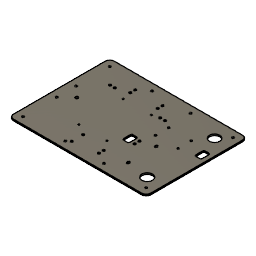
layer3_plate_v0_1 (Autodesk Fusion 360 design; units mm, degrees)
part number: 2026-05-30-19-40-51-836
Autodesk Fusion 360 part; units mm, degrees
box "长方体基本要素1" add length 209.6 width 285 height 3 placed x (0, 0, 1) y (1, 0, 0) z (0, 1, 0) at (0, 0, 0)
sketch "草图2" plane through (0, 3, 0) normal (0, 1, 0) x (-1, 0, 0)
  line L0 (0, 209.6) -> (-285, 209.6)
  line L1 (-285, 209.6) -> (-285, 0)
  line L2 (-285, 0) -> (0, 0)
  line L3 (0, 0) -> (0, 209.6)
  line L4 (-285, 104.8) -> (0, 104.8) construction
  line L5 (-142.5, 0) -> (-142.5, 209.6) construction
  circle A0 centre (-252.0096, 174.6) radius 11.05
  circle A1 centre (-252.0096, 35) radius 10.68
  circle A2 centre (-252.0096, 35) radius 14.275
  line L6 (-252.0096, 189.6) -> (-265, 182.1)
  line L7 (-265, 182.1) -> (-265, 167.1)
  line L8 (-265, 167.1) -> (-252.0096, 159.6)
  line L9 (-252.0096, 159.6) -> (-239.0192, 167.1)
  line L10 (-239.0192, 167.1) -> (-239.0192, 182.1)
  line L11 (-239.0192, 182.1) -> (-252.0096, 189.6)
  line L12 (-70.6, 54.8) -> (-148.4, 54.8)
  line L13 (-149, 55.4) -> (-149, 154.2)
  line L14 (-148.4, 154.8) -> (-70.6, 154.8)
  line L15 (-70, 154.2) -> (-70, 55.4)
  line L16 (-70, 54.8) -> (-149, 154.8) construction
  line L17 (-149, 54.8) -> (-70, 154.8) construction
  line L18 (-179, 59.87) -> (-239.07, 59.87)
  line L19 (-239.07, 59.87) -> (-239.07, 94.8)
  line L20 (-239.07, 94.8) -> (-179, 94.8)
  line L21 (-179, 94.8) -> (-179, 59.87)
  line L22 (0, 72.3) -> (-30, 72.3)
  line L23 (-30, 72.3) -> (-30, 137.3)
  line L24 (-30, 137.3) -> (0, 137.3)
  arc A3 (-70.6, 54.8) -> (-70, 55.4) centre (-70.6, 55.4) ccw
  arc A4 (-149, 55.4) -> (-148.4, 54.8) centre (-148.4, 55.4) ccw
  arc A5 (-70, 154.2) -> (-70.6, 154.8) centre (-70.6, 154.2) ccw
  arc A6 (-148.4, 154.8) -> (-149, 154.2) centre (-148.4, 154.2) ccw
  circle A7 centre (-270, 194.6) radius 2.15
  circle A8 centre (-270, 15) radius 2.15
  circle A9 centre (-15, 15) radius 2.15
  circle A10 centre (-15, 194.6) radius 2.15
  circle A11 centre (-182.5, 15) radius 2.15
  circle A12 centre (-102.5, 15) radius 2.15
  circle A13 centre (-102.5, 194.6) radius 2.15
  circle A14 centre (-182.5, 194.6) radius 2.15
  line L25 (-15, 72.3) -> (-15, 137.3) construction
  circle A15 centre (-15, 84.8) radius 2.15
  circle A16 centre (-15, 124.8) radius 2.15
  line L26 (-109.5, 54.8) -> (-109.5, 154.8) construction
  circle A17 centre (-87, 58.8) radius 1.6
  circle A18 centre (-145, 58.8) radius 1.6
  circle A19 centre (-87, 150.8) radius 1.6
  circle A20 centre (-145, 150.8) radius 1.6
  circle A21 centre (-232.375, 63.695) radius 1.99
  line L27 (-209.035, 59.87) -> (-209.035, 94.8) construction
  line L28 (-239.07, 77.335) -> (-179, 77.335) construction
  circle A22 centre (-232.375, 90.975) radius 1.99
  circle A23 centre (-185.695, 63.695) radius 1.99
  circle A24 centre (-185.695, 90.975) radius 1.99
  line L29 (-273, 68.335) -> (-265, 68.335)
  line L30 (-263, 70.335) -> (-263, 84.335)
  line L31 (-265, 86.335) -> (-273, 86.335)
  line L32 (-275, 84.335) -> (-275, 70.335)
  arc A25 (-265, 68.335) -> (-263, 70.335) centre (-265, 70.335) ccw
  arc A26 (-275, 70.335) -> (-273, 68.335) centre (-273, 70.335) ccw
  arc A27 (-263, 84.335) -> (-265, 86.335) centre (-265, 84.335) ccw
  arc A28 (-273, 86.335) -> (-275, 84.335) centre (-273, 84.335) ccw
  circle A29 centre (-109.5, 164.8) radius 1.75
  circle A30 centre (-109.5, 188.3) radius 1.75
  line L33 (-109.5, 188.3) -> (-109.5, 164.8) construction
  line L34 (-109.5, 176.55) -> (-126.71, 176.55) construction
  circle A31 centre (-169, 54.8) radius 1.75
  circle A32 centre (-159, 54.8) radius 1.75
  circle A33 centre (-139.6536, 30.484) radius 1.75
  circle A34 centre (-139.6536, 40.484) radius 1.75
  circle A35 centre (-82.9945, 30.484) radius 1.75
  circle A36 centre (-82.9945, 40.484) radius 1.75
  line L35 (-139.6536, 30.484) -> (-139.6536, 40.484) construction
  line L36 (-138.8486, 35.484) -> (-115.3178, 35.484) construction
  circle A37 centre (-58.3945, 48.0031) radius 1.75
  circle A38 centre (-48.3945, 48.0031) radius 1.75
  circle A39 centre (-264, 157.9214) radius 1.75
  circle A40 centre (-252.0096, 174.6) radius 22.75
  line L37 (-273, 68.335) -> (-265, 68.335)
  line L38 (-275, 84.335) -> (-275, 70.335)
  line L39 (-265, 86.335) -> (-273, 86.335)
  line L40 (-263, 70.335) -> (-263, 84.335)
  arc A41 (-273, 86.335) -> (-275, 84.335) centre (-273, 84.335) ccw
  arc A42 (-265, 68.335) -> (-263, 70.335) centre (-265, 70.335) ccw
  arc A43 (-263, 84.335) -> (-265, 86.335) centre (-265, 84.335) ccw
  arc A44 (-275, 70.335) -> (-273, 68.335) centre (-273, 70.335) ccw
  circle A45 centre (-158.9706, 171.55) radius 1.75
  circle A46 centre (-158.9706, 181.55) radius 1.75
  line L41 (-222.2263, 163.8539) -> (-190.2263, 163.8539)
  line L42 (-190.2263, 163.8539) -> (-190.2263, 113.8539)
  line L43 (-190.2263, 113.8539) -> (-222.2263, 113.8539)
  line L44 (-222.2263, 113.8539) -> (-222.2263, 163.8539)
  line L45 (-206.2263, 163.8539) -> (-206.2263, 166.8539) construction
  line L46 (-206.2263, 166.8539) -> (-206.2263, 168.7439) construction
  line L47 (-208.3763, 166.8539) -> (-208.3763, 168.7439)
  line L48 (-204.0763, 168.7439) -> (-204.0763, 166.8539)
  arc A47 (-204.0763, 168.7439) -> (-208.3763, 168.7439) centre (-206.2263, 168.7439) ccw
  arc A48 (-208.3763, 166.8539) -> (-204.0763, 166.8539) centre (-206.2263, 166.8539) ccw
  line L49 (-222.2263, 138.8539) -> (-190.2263, 138.8539) construction
  arc A49 (-204.0763, 110.8539) -> (-208.3763, 110.8539) centre (-206.2263, 110.8539) ccw
  line L50 (-206.2263, 110.8539) -> (-206.2263, 108.9639) construction
  line L51 (-208.3763, 110.8539) -> (-208.3763, 108.9639)
  arc A50 (-208.3763, 108.9639) -> (-204.0763, 108.9639) centre (-206.2263, 108.9639) ccw
  line L52 (-204.0763, 108.9639) -> (-204.0763, 110.8539)
  line L53 (-161, 113.8539) -> (-169, 113.8539)
  line L54 (-171, 115.8539) -> (-171, 129.8539)
  line L55 (-169, 131.8539) -> (-161, 131.8539)
  line L56 (-159, 129.8539) -> (-159, 115.8539)
  arc A51 (-161, 113.8539) -> (-159, 115.8539) centre (-161, 115.8539) ccw
  arc A52 (-171, 115.8539) -> (-169, 113.8539) centre (-169, 115.8539) ccw
  arc A53 (-169, 131.8539) -> (-171, 129.8539) centre (-169, 129.8539) ccw
  arc A54 (-159, 129.8539) -> (-161, 131.8539) centre (-161, 129.8539) ccw
  line L57 (-171, 122.8539) -> (-159, 122.8539) construction
  circle A55 centre (-179.3475, 117.8539) radius 1.75
  circle A56 centre (-179.3475, 127.8539) radius 1.75
  line L58 (-124, 124.8) -> (-144, 124.8)
  line L59 (-144, 124.8) -> (-144, 144.8)
  line L60 (-144, 144.8) -> (-124, 144.8)
  line L61 (-124, 144.8) -> (-124, 124.8)
  circle A57 centre (-125.75, 15) radius 3.25
  circle A58 centre (-125.75, 194.6) radius 3.25
  point P0 (-252.0096, 174.6)
  point P1 (-109.5, 104.8)
  point P2 (-182.5, 194.6)
  point P3 (-275, 68.335)
  point P4 (-263, 68.335)
  point P5 (-275, 86.335)
  point P6 (-275, 68.335)
  point P7 (-263, 68.335)
  point P8 (-275, 86.335)
  point P9 (-159, 113.8539)
  point P10 (-171, 113.8539)
  point P11 (-159, 131.8539)
  dimension "d8" = 22.1
  dimension "d9" = 21.36
  dimension "d10" = 28.55
  dimension "d11" = 15
  dimension "d12" = 20
  dimension "d14" = 79
  dimension "d15" = 100
  dimension "d18" = 34.93
  dimension "d19" = 60.07
  dimension "d20" = 30
  dimension "d21" = 65
  dimension "d22" = 40
  dimension "d33" = 0.6
  dimension "d34" = 0.6
  dimension "d35" = 0.6
  dimension "d36" = 0.6
  dimension "d47" = 4.3
  dimension "d48" = 15
  dimension "d49" = 15
  dimension "d50" = 4.3
  dimension "d51" = 15
  dimension "d52" = 80
  dimension "d53" = 4.3
  dimension "d54" = 40
  dimension "d55" = 3.2
  dimension "d56" = 4
  dimension "d57" = 3.2
  dimension "d58" = 4
  dimension "d59" = 4
  dimension "d60" = 58
  dimension "d61" = 3.98
  dimension "d62" = 27.28
  dimension "d63" = 46.68
  dimension "d75" = 12
  dimension "d76" = 18
  dimension "d79" = 10
  dimension "d81" = 2
  dimension "d82" = 2
  dimension "d83" = 2
  dimension "d84" = 2
  dimension "d99" = 35
  dimension "d100" = 3.5
  dimension "d101" = 3.5
  dimension "d102" = 23.5
  dimension "d103" = 10
  dimension "d107" = 3.5
  dimension "d108" = 10
  dimension "d109" = 10
  dimension "d110" = 3.5
  dimension "d111" = 10
  dimension "d112" = 10
  dimension "d113" = 3.5
  dimension "d114" = 10
  dimension "d123" = 30
  dimension "d124" = 45.5
  dimension "d144" = 12
  dimension "d145" = 18
  dimension "d146" = 2
  dimension "d147" = 2
  dimension "d148" = 2
  dimension "d149" = 2
  dimension "d185" = 3.5
  dimension "d186" = 3.5
  dimension "d187" = 10
  dimension "d210" = 32
  dimension "d211" = 50
  dimension "d212" = 3
  dimension "d214" = 1.89
  dimension "d215" = 2.15
  dimension "d218" = 12
  dimension "d219" = 18
  dimension "d220" = 2
  dimension "d223" = 10
  dimension "d224" = 3.5
  dimension "d225" = 3.5
  dimension "d226" = 10
  dimension "d227" = 9
  dimension "d248" = 20
  dimension "d249" = 20
  dimension "d250" = 10
  dimension "d251" = 5
  dimension "d252" = 6.5
  dimension "d253" = 23.25
  dimension "d254" = 15
  constraint midpoint L1 L4.start
  constraint midpoint L3 L4.end
  constraint midpoint L2 L5.start
  constraint midpoint L0 L5.end
  constraint concentric A1 A2
  constraint coincident P0 A0.centre
  constraint symmetric L4 P0 A1.centre
  constraint parallel L1 L7
  constraint horizontal L12
  constraint perpendicular L12 L13
  constraint parallel L12 L14
  constraint parallel L13 L15
  constraint coincident L16 P1
  constraint coincident L17 P1
  constraint horizontal L18
  constraint vertical L19
  constraint horizontal L20
  constraint vertical L21
  constraint coincident L4 P1
  constraint coincident L3 L22.start
  constraint perpendicular L3 L22
  constraint perpendicular L4 L23
  constraint coincident L3 L24.end
  constraint perpendicular L3 L24
  constraint symmetric L4 L22 L24
  constraint coincident L16.start L15
  constraint coincident L16.start L12
  constraint tangent L15 A3
  constraint tangent L12 A3
  constraint coincident L17.start L12
  constraint coincident L17.start L13
  constraint tangent L12 A4
  constraint tangent L13 A4
  constraint coincident L17.end L14
  constraint coincident L17.end L15
  constraint tangent L14 A5
  constraint tangent L15 A5
  constraint coincident L16.end L14
  constraint coincident L16.end L13
  constraint tangent L14 A6
  constraint tangent L13 A6
  constraint symmetric L4 A7 A8
  constraint symmetric L5 A7 A10
  constraint symmetric L5 A8 A9
  constraint symmetric L5 A11 A12
  constraint symmetric L4 A11.centre P2
  constraint symmetric L4 A12 A13
  constraint symmetric L4 A11 A14
  constraint midpoint L22 L25.start
  constraint midpoint L24 L25.end
  constraint coincident L25 A15.centre
  constraint symmetric L4 A15 A16
  constraint midpoint L12 L26.start
  constraint midpoint L14 L26.end
  constraint symmetric L4 A17 A19
  constraint symmetric L4 A18 A20
  constraint midpoint L18 L27.start
  constraint midpoint L20 L27.end
  constraint midpoint L19 L28.start
  constraint midpoint L21 L28.end
  constraint symmetric A21 L28 A22
  constraint symmetric A21 L27 A23
  constraint symmetric L27 A22 A24
  constraint horizontal L29
  constraint vertical L30
  constraint horizontal L31
  constraint vertical L32
  constraint symmetric L28 L29 L31
  constraint coincident P7 L30
  constraint tangent L30 A25
  constraint tangent L29 A25
  constraint coincident P6 L32
  constraint tangent L32 A26
  constraint tangent L29 A26
  constraint tangent L31 A27
  constraint tangent L30 A27
  constraint coincident P8 L31
  constraint coincident P8 L32
  constraint tangent L31 A28
  constraint tangent L32 A28
  constraint vertical A29.centre A30.centre
  constraint coincident A30.centre L33.start
  constraint coincident A29.centre L33.end
  constraint midpoint L33 L34.start
  constraint perpendicular L33 L34
  constraint equal A31 A32
  constraint horizontal L12.end A32.centre
  constraint horizontal A31.centre A32.centre
  constraint equal A35 A36
  constraint equal A34 A36
  constraint equal A33 A36
  constraint vertical A33.centre A34.centre
  constraint vertical A35.centre A36.centre
  constraint coincident A33.centre L35.start
  constraint coincident A34.centre L35.end
  constraint perpendicular L35 L36
  constraint symmetric A33.centre A34.centre L36
  constraint symmetric A35.centre A36.centre L36
  constraint equal A37 A38
  constraint horizontal A37.centre A38.centre
  constraint concentric A0 A40
  constraint horizontal L37
  constraint vertical L40
  constraint horizontal L39
  constraint vertical L38
  constraint coincident P7 L40
  constraint tangent L40 A42
  constraint tangent L37 A42
  constraint coincident P6 L38
  constraint tangent L38 A44
  constraint tangent L37 A44
  constraint tangent L39 A43
  constraint tangent L40 A43
  constraint coincident P8 L39
  constraint coincident P8 L38
  constraint tangent L39 A41
  constraint tangent L38 A41
  constraint vertical A45.centre A46.centre
  constraint symmetric L34 A45.centre A46.centre
  constraint horizontal L41
  constraint vertical L42
  constraint horizontal L43
  constraint vertical L44
  constraint midpoint L41 L45.start
  constraint perpendicular L41 L45
  constraint coincident L45.end L46.start
  constraint parallel L45 L46
  constraint coincident L46.end A47.centre
  constraint equal A47 A48
  constraint tangent L48 A48
  constraint tangent L48 A47
  constraint tangent L47 A48
  constraint tangent L47 A47
  constraint midpoint L44 L49.start
  constraint midpoint L42 L49.end
  constraint symmetric L45.end L49 A49.centre
  constraint symmetric L46.end L49 L50.end
  constraint symmetric L47.start L49 A49.end
  constraint symmetric L47.end L49 L51.end
  constraint symmetric L48.start L49 A50.end
  constraint symmetric L48.end L49 A49.start
  constraint symmetric A47 L49 A50
  constraint symmetric A48 L49 A49
  constraint horizontal L53
  constraint vertical L54
  constraint horizontal L55
  constraint vertical L56
  constraint coincident P9 L56
  constraint coincident P9 L53
  constraint tangent L56 A51
  constraint tangent L53 A51
  constraint coincident P10 L54
  constraint coincident P10 L53
  constraint tangent L54 A52
  constraint tangent L53 A52
  constraint tangent L55 A53
  constraint tangent L54 A53
  constraint equal A52 A53
  constraint coincident P11 L55
  constraint coincident P11 L56
  constraint tangent L55 A54
  constraint tangent L56 A54
  constraint equal A51 A52
  constraint equal A51 A54
  constraint midpoint L54 L57.start
  constraint midpoint L56 L57.end
  constraint symmetric L57 A55.centre A56.centre
  constraint horizontal L58
  constraint vertical L59
  constraint horizontal L60
  constraint vertical L61
  constraint symmetric L4 A57 A58
  measures "d8" diameter of A0
  measures "d9" diameter of A1
  measures "d10" diameter of A2
  measures "d11" distance of L6.start L10.end
  measures "d12" distance of L1 L7
  measures "d14" distance of L16.end L17.end
  measures "d15" distance of L17.start L16.end
  measures "d18" distance of L18.start L20.end
  measures "d19" distance of L18.start L18.end
  measures "d20" distance of L22.start L22.end
  measures "d21" distance of L22.end L23.end
  measures "d22" distance of L15 L23
  measures "d33" radius of A3
  measures "d34" radius of A4
  measures "d35" radius of A5
  measures "d36" radius of A6
  measures "d47" diameter of A7
  measures "d48" distance of L0 A7.centre
  measures "d49" distance of L1 A7.centre
  measures "d50" diameter of A11
  measures "d51" distance of L2 A11.centre
  measures "d52" distance of A11.centre A12.centre
  measures "d53" diameter of A15
  measures "d54" distance of A15.centre A16.centre
  measures "d55" diameter of A17
  measures "d56" distance of L12 A17.centre
  measures "d57" diameter of A18
  measures "d58" distance of L12 A18.centre
  measures "d59" distance of L13 A18.centre
  measures "d60" distance of A17.centre A18.centre
  measures "d61" diameter of A21
  measures "d62" distance of A21.centre A22.centre
  measures "d63" distance of A21.centre A23.centre
  measures "d75" distance of P6 P7
  measures "d76" distance of P6 P8
  measures "d79" distance of L1 L32
  measures "d81" radius of A25
  measures "d82" radius of A26
  measures "d83" radius of A27
  measures "d84" radius of A28
  measures "d99" distance of L0 P0
  measures "d100" diameter of A29
  measures "d101" diameter of A30
  measures "d102" vertical distance of A29.centre A30.centre
  measures "d103" distance of L14 A29.centre
  measures "d107" diameter of A31
  measures "d108" distance of A31.centre A32.centre
  measures "d109" distance of L21 A31.centre
  measures "d110" diameter of A36
  measures "d111" distance of A33.centre A34.centre
  measures "d112" distance of A35.centre A36.centre
  measures "d113" diameter of A37
  measures "d114" distance of A37.centre A38.centre
  measures "d123" distance of L13 L21
  measures "d124" diameter of A40
  measures "d144" distance of P6 P7
  measures "d145" distance of P6 P8
  measures "d146" radius of A42
  measures "d147" radius of A44
  measures "d148" radius of A43
  measures "d149" radius of A41
  measures "d185" diameter of A45
  measures "d186" diameter of A46
  measures "d187" distance of A45.centre A46.centre
  measures "d210" distance of L41.start L41.end
  measures "d211" distance of L41.start L43.end
  measures "d212" distance of L45.start L45.end
  measures "d214" distance of L45.end L46.end
  measures "d215" radius of A48
  measures "d218" distance of P9 P10
  measures "d219" distance of P9 P11
  measures "d220" radius of A51
  measures "d223" distance of L13 L56
  measures "d224" diameter of A55
  measures "d225" diameter of A56
  measures "d226" distance of A55.centre A56.centre
  measures "d227" distance of L43 L57
  measures "d248" distance of L58.start L58.end
  measures "d249" distance of L58.start L60.end
  measures "d250" distance of L14 L60
  measures "d251" distance of L13 L59
  measures "d252" diameter of A57
  measures "d253" distance of L13 A57.centre
  measures "d254" distance of L2 A57.centre
extrude "拉伸1" cut sketch "草图2" against normal blind 33 contours A0
extrude "拉伸2" cut sketch "草图2" against normal blind 45 contours A1
extrude "拉伸3" cut sketch "草图2" against normal blind 3 contours A7 | A8 | A9 | A10 | A11 | A12 | A13 | A14 | A15 | A16 | A17 | A19 | A20 | A21 | A22 | A23 | A24
sketch "草图3" plane through (0, 0, 0) normal (0, -1, 0) x (1, 0, 0)
  circle A0 centre (252.0096, 35) radius 10.68
  circle A1 centre (252.0096, 174.6) radius 11.05
  line L0 (285, 209.6) -> (0, 209.6)
  line L1 (0, 209.6) -> (0, 0)
  line L2 (0, 0) -> (285, 0)
  line L3 (285, 0) -> (285, 209.6)
  line L4 (0, 104.8) -> (285, 104.8) construction
  line L5 (30, 116.15) -> (45.664, 116.15)
  line L6 (45.664, 116.15) -> (45.664, 93.45)
  line L7 (45.664, 93.45) -> (30, 93.45)
  line L8 (30, 93.45) -> (30, 116.15)
  circle A2 centre (182.5, 194.6) radius 2.15
  circle A3 centre (182.5, 15) radius 2.15
  circle A4 centre (232.375, 63.695) radius 1.99
  circle A5 centre (87, 58.8) radius 1.6
  circle A6 centre (87, 150.8) radius 1.6
  circle A7 centre (15, 124.8) radius 2.15
  circle A8 centre (102.5, 15) radius 2.15
  circle A9 centre (185.695, 90.975) radius 1.99
  circle A10 centre (270, 15) radius 2.15
  circle A11 centre (185.695, 63.695) radius 1.99
  circle A12 centre (15, 194.6) radius 2.15
  circle A13 centre (102.5, 194.6) radius 2.15
  circle A14 centre (15, 84.8) radius 2.15
  circle A15 centre (145, 150.8) radius 1.6
  circle A16 centre (15, 15) radius 2.15
  circle A17 centre (232.375, 90.975) radius 1.99
  circle A18 centre (270, 194.6) radius 2.15
  circle A19 centre (36.25, 104.8) radius 2.9
  dimension "d42" = 22.7
  dimension "d43" = 15.664
  dimension "d46" = 30
  dimension "d71" = 6.25
  dimension "d72" = 5.8
  constraint midpoint L1 L4.start
  constraint midpoint L3 L4.end
  constraint horizontal L5
  constraint vertical L6
  constraint horizontal L7
  constraint vertical L8
  constraint symmetric L4 L5 L7
  constraint coincident L4 A19.centre
  measures "d42" distance of L5.start L7.end
  measures "d43" distance of L6.end L7.end
  measures "d46" distance of L1 L8
  measures "d71" distance of L8 A19.centre
  measures "d72" diameter of A19
extrude "拉伸17" cut sketch "草图3" against normal blind 3 contours A19
extrude "拉伸18" cut sketch "草图2" against normal blind 3 contours L29 L30 L31 L32 A25 A26 A27 A28 L37 L38 L39 L40 A41 A42 A43 A44 | A29 | A30 | A31 | A32 | A33 | A34 | A35 | A36 | A37 | A38 | A45 | A46
extrude "拉伸19" cut sketch "草图2" against normal blind 3 contours A18
extrude "拉伸20" cut sketch "草图2" against normal blind 3 contours L47 L48 A47 A48 | A49 L51 A50 L52
extrude "拉伸21" cut sketch "草图2" against normal blind 3 contours L53 L54 L55 L56 A51 A52 A53 A54 | A55 | A56
fillet "圆角9" radius 10 1 edges at (0, 1.5, 0)
fillet "圆角10" radius 10 1 edges at (0, 1.5, 209.6)
fillet "圆角11" radius 10 1 edges at (285, 1.5, 209.6)
fillet "圆角12" radius 10 1 edges at (285, 1.5, 0)
fillet "圆角13" radius 0.5 16 edges at (275, 3, 77.335) (274.4142, 3, 85.7492) (269, 3, 86.335) (263.5858, 3, 85.7492) (263, 3, 77.335) (263.5858, 3, 68.9208) (269, 3, 68.335) (274.4142, 3, 68.9208) (263, 0, 77.335) (263.5858, 0, 85.7492) (269, 0, 86.335) (274.4142, 0, 85.7492) (275, 0, 77.335) (274.4142, 0, 68.9208) (269, 0, 68.335) (263.5858, 0, 68.9208)
fillet "圆角14" radius 0.5 38 edges at (171, 3, 122.8539) (170.4142, 3, 131.2681) (165, 3, 131.8539) (159.5858, 3, 131.2681) (159, 3, 122.8539) (159.5858, 3, 114.4397) (165, 3, 113.8539) (170.4142, 3, 114.4397) (159, 0, 122.8539) (159.5858, 0, 131.2681) (165, 0, 131.8539) (170.4142, 0, 131.2681) (171, 0, 122.8539) (170.4142, 0, 114.4397) (165, 0, 113.8539) (159.5858, 0, 114.4397) (160.6316, 3, 55.4328) (160.6316, 0, 54.1672) (170.6316, 0, 54.1672) (141.2852, 3, 41.1168) (141.2852, 0, 39.8512) (141.2852, 3, 31.1168) (141.2852, 0, 29.8512) (84.626, 0, 39.8512) (84.626, 3, 41.1168) (84.626, 0, 29.8512) (84.626, 3, 31.1168) (50.0261, 0, 47.3703) (60.0261, 0, 47.3703) (60.0261, 3, 48.6359) (111.1316, 3, 188.9328) (111.1316, 0, 187.6672) (111.1316, 0, 164.1672) (111.1316, 3, 165.4328) (160.6021, 3, 172.1828) (160.6021, 0, 170.9172) (160.6021, 0, 180.9172) (160.6021, 3, 182.1828) 1 faces at (46.6467, 1, 47.9159)
fillet "圆角15" radius 0.5 1 edges at (170.6316, 3, 55.4328)
fillet "圆角16" radius 0.5 4 edges at (180.9791, 3, 118.4867) (180.9791, 0, 117.2211) (180.9791, 3, 128.4867) (180.9791, 0, 127.2211)
fillet "圆角17" radius 0.5 16 edges at (2.9289, 3, 2.9289) (0, 3, 104.8) (2.9289, 3, 206.6711) (142.5, 3, 209.6) (282.0711, 3, 206.6711) (285, 3, 104.8) (282.0711, 3, 2.9289) (142.5, 3, 0) (282.0711, 0, 2.9289) (285, 0, 104.8) (282.0711, 0, 206.6711) (142.5, 0, 209.6) (2.9289, 0, 206.6711) (0, 0, 104.8) (2.9289, 0, 2.9289) (142.5, 0, 0)
equation "d59 = ( 2.794 / 2 ) * 1 mm + 2.603 mm"
equation "d253 = 20 mm + 3.25 mm"
